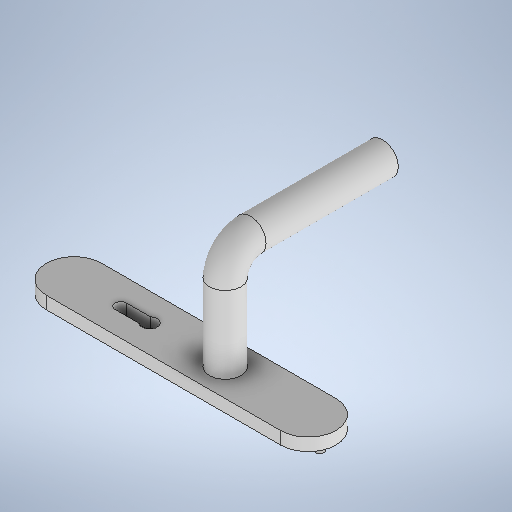
# Autodesk Inventor part: garnitur_lang
Saved by Autodesk Inventor 2025.1 (Build 291241000, 241)
## iProperties
Created: 2024-08-07
Part Number: garnitur_lang
Material: Generisch
Document SubType Name: Modeling
Designer: ffogue
Density: 1 g/cm^3
Appearance: Vorgabe
Author: ffogue
Autodesk Inventor part; units mm, degrees
ref_plane "YZ Plane" through (0, 0, 0) normal (1, 0, 0) x (0, 1, 0)
ref_plane "XZ Plane" through (0, 0, 0) normal (0, 1, 0) x (-1, 0, 0)
sketch "Sketch1" plane through (0, 0, 0) normal (0, 0, 1) x (1, 0, 0)
  circle A0 centre (0, 0) radius 12.5
  dimension "d0" = 25
  constraints: 1 centre point, 1 coincident
  measures "d0" diameter of A0
sketch "Sketch2" plane through (0, 0, 0) normal (1, 0, 0) x (0, 1, 0)
  line L0 (0, 0) -> (0, 61)
  arc A0 (20, 81) -> (0, 61) centre (20, 61) ccw
  line L1 (20, 81) -> (125, 81)
  dimension "d1" = 61
  dimension "d30" = 105
  dimension "d31" = 20
  constraints: 4 end point, 2 point on circle, 2 tangent, 1 centre point, 1 horizontal, 1 vertical
  measures "d1" distance of L0.start L0.end
  measures "d30" distance of L1.start L1.end
  measures "d31" radius of A0
ref_plane "Work Plane1" through (0, 0, 61) normal (0, 0, 1) x (1, 0, 0)
sweep "Sweep2" add profiles "Sketch1" path "Sketch2"
sketch "Sketch4" plane through (0, 0, 0) normal (0, 0, -1) x (-1, 0, 0)
  line L0 (-66, 0) -> (120, 0) construction
  line L1 (-66, 22) -> (120, 22)
  line L2 (120, -22) -> (-66, -22)
  arc A0 (-66, 22) -> (-66, -22) centre (-66, 0) ccw
  arc A1 (120, -22) -> (120, 22) centre (120, 0) ccw
  circle A2 centre (0, 0) radius 12.5 projected
  point P0 (27, 0)
  point P1 (27, 0)
  point P2 (142, 0)
  point P3 (-88, 0)
  dimension "d10" = 44
  dimension "d12" = 88
  dimension "d13" = 230
  constraints: 8 end point, 6 point on circle, 4 tangent, 2 centre point, 1 coincident, 1 horizontal, 1 horizontal alignment, 1 midpoint, 1 parallel
  measures "d10" distance between parallel lines of L2 L1
  measures "d12" distance of point (-88, 0) A2.centre
  measures "d13" distance of point (142, 0) point (-88, 0)
extrude "Extrusion1" add sketch "Sketch4" along normal blind 10 contours L1 A1 L2 A0 | A2
sketch "Sketch5" plane through (0, 0, -10) normal (0, 0, -1) x (-1, 0, 0)
  circle A0 centre (-75, 0) radius 3.5
  circle A1 centre (21.5, 0) radius 3.5
  circle A2 centre (112, 0) radius 3.5
  circle A3 centre (0, 0) radius 12.5 projected
  dimension "d16" = 7
  dimension "d17" = 21.5
  dimension "d18" = 75
  dimension "d19" = 90.5
  constraints: 3 centre point, 3 horizontal alignment, 2 equal radius
  measures "d16" diameter of A0
  measures "d17" distance of A1.centre point (0, 0)
  measures "d18" distance of A0.centre point (0, 0)
  measures "d19" distance of A2.centre A1.centre
extrude "Extrusion2" add sketch "Sketch5" along normal blind 10 contours A0 | A1 | A2
sketch "Sketch6" plane through (0, 0, 0) normal (0, 0, 1) x (1, 0, 0)
  arc A0 (-63.9686, -4.5) -> (-63.9686, 4.5) centre (-60, 0) ccw
  circle A1 centre (0, 0) radius 12.5 projected
  line L0 (-63.9686, 4.5) -> (-83, 4.5)
  arc A2 (-83, 4.5) -> (-83, -4.5) centre (-83, 0) ccw
  line L1 (-83, -4.5) -> (-63.9686, -4.5)
  arc A3 (-120, 22) -> (-120, -22) centre (-120, 0) ccw projected
  point P0 (-142, 0)
  dimension "d22" = 12
  dimension "d23" = 60
  dimension "d24" = 4.5
  dimension "d25" = 23
  constraints: 5 point on circle, 4 end point, 2 centre point, 2 horizontal alignment, 2 tangent, 1 horizontal, 1 parallel
  measures "d22" diameter of A0
  measures "d23" distance of A0.centre A1.centre
  measures "d24" radius of A2
  measures "d25" distance of A2.centre A0.centre
extrude "Extrusion3" cut sketch "Sketch6" against normal blind 10 contours L1 A2 L0 A0
body "Solid2"
